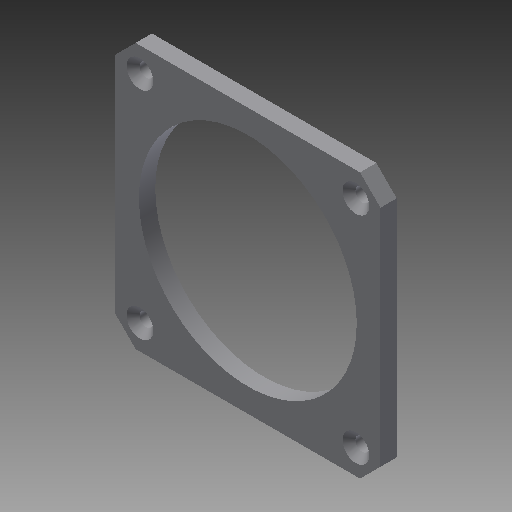
# Autodesk Inventor part: Крышка
Saved by Autodesk Inventor 2022 (Build 260153000, 153)
## iProperties
RuleStatus: InUse
Part Number: Крышка
Checked By: Якушев
Engr Approved By: Малов
Material: По умолчанию1
Document SubType Name: Modeling
Mfg Approved By: Судаков
Designer: Смирнов
Density: 1 g/cm^3
Appearance: По умолчанию1
Mass: 7.52445 g
Surface Area: 56.0651 cm^2
Volume: 7.52445 cm^3
AfterMaterialChange0: Материал
BeforeDocSave0: Материал
AfterAnyiPropertyChange0: Материал
Материал: По умолчанию1
Author: Смирнов
Title: Крышка
Autodesk Inventor part; units mm, degrees
ref_plane "YZ Plane" through (0, 0, 0) normal (1, 0, 0) x (0, 1, 0)
ref_plane "XZ Plane" through (0, 0, 0) normal (0, 1, 0) x (-1, 0, 0)
ref_plane "РабПлоскость1" through (0, 0, 75.2) normal (0, 0, 1) x (1, 0, 0)
sketch "Эскиз1" plane through (0, 0, 75.2) normal (0, 0, 1) x (1, 0, 0)
  circle A0 centre (26.4645, -26.4645) radius 1.95 construction
  circle A1 centre (-26.4645, 26.4645) radius 1.95 construction
  circle A2 centre (26.4645, 26.4645) radius 1.95 construction
  circle A3 centre (-26.4645, -26.4645) radius 1.95 construction
  circle A4 centre (15.35, -15.35) radius 1.7 construction
  circle A5 centre (-15.35, 15.35) radius 1.7 construction
  circle A6 centre (15.35, 15.35) radius 1.7 construction
  circle A7 centre (-15.35, -15.35) radius 1.7 construction
  line L0 (-32.5, 27.5) -> (-32.5, -27.5) projected
  line L1 (-27.5, 32.5) -> (-32.5, 27.5) projected
  line L2 (27.5, 32.5) -> (-27.5, 32.5) projected
  line L3 (32.5, 27.5) -> (27.5, 32.5) projected
  line L4 (32.5, -27.5) -> (32.5, 27.5) projected
  line L5 (27.5, -32.5) -> (32.5, -27.5) projected
  line L6 (-27.5, -32.5) -> (27.5, -32.5) projected
  line L7 (-32.5, -27.5) -> (-27.5, -32.5) projected
  circle A8 centre (0, 0) radius 11.5 construction
  circle A9 centre (0, 0) radius 26.7 projected
  point P0 (0, 0)
extrude "Выдавливание1" add sketch "Эскиз1" along normal blind 4
sketch "Эскиз2" plane through (0, 0, 79.2) normal (0, 0, 1) x (1, 0, 0)
  circle A0 centre (26.4645, 26.4645) radius 2.25 projected
  circle A1 centre (26.4645, -26.4645) radius 2.25 projected
  circle A2 centre (-26.4645, -26.4645) radius 2.25 projected
  circle A3 centre (-26.4645, 26.4645) radius 1.95 projected
hole "Отверстие1" at (26.4645, 26.4645, 79.2) at (-26.4645, 26.4645, 79.2) at (26.4645, -26.4645, 79.2) at (-26.4645, -26.4645, 79.2) direction (0, 0, -1) diameter 3.4 end through all countersink diameter 6.6 countersink angle 90 clearance for "с потайной головкой ГОСТ 12876-67" size "M3" standard "ГОСТ"
